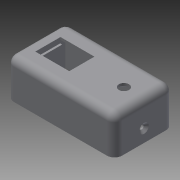
# Autodesk Inventor part: obudowa - timer- front
Saved by Autodesk Inventor 2014 (Build 180170000, 170)
## iProperties
Created: 2018-02-28
Part Number: obudowa - timer- front
Material: Generic
Document SubType Name: Modeling
Designer: HP820
Density: 1 g/cm^3
Appearance: Default
Author: HP820
Autodesk Inventor part; units mm, degrees
ref_plane "YZ Plane" through (0, 0, 0) normal (1, 0, 0) x (0, 1, 0)
ref_plane "XZ Plane" through (0, 0, 0) normal (0, 1, 0) x (-1, 0, 0)
ref_plane "XY Plane" through (0, 0, 0) normal (0, 0, 1) x (1, 0, 0)
sketch "Sketch1" plane through (0, 0, 0) normal (0, 0, 1) x (1, 0, 0)
  line L0 (-40, 20.5) -> (40, 20.5)
  line L1 (40, 20.5) -> (40, -20.5)
  line L2 (40, -20.5) -> (-40, -20.5)
  line L3 (-40, -20.5) -> (-40, 20.5)
  line L4 (-40, 20.5) -> (40, -20.5) construction
  line L5 (40, 20.5) -> (-40, -20.5) construction
  line L6 (-43, 23.5) -> (43, 23.5)
  line L7 (43, 23.5) -> (43, -23.5)
  line L8 (43, -23.5) -> (-43, -23.5)
  line L9 (-43, -23.5) -> (-43, 23.5)
  line L10 (-43, 23.5) -> (43, -23.5) construction
  line L11 (43, 23.5) -> (-43, -23.5) construction
  point P0 (0, 0)
  dimension "d0" = 80
  dimension "d1" = 41
  dimension "d2" = 86
  dimension "d3" = 47
  constraints: 24 end point, 4 midpoint, 4 parallel, 2 horizontal, 2 perpendicular
  measures "d0" distance of L1.end L2.end
  measures "d1" distance of L0.end L1.end
  measures "d2" distance of L7.end L8.end
  measures "d3" distance of L6.end L7.end
extrude "Extrusion1" add sketch "Sketch1" against normal blind 30
sketch "Sketch2" plane through (0, 0, 0) normal (0, 0, 1) x (1, 0, 0)
  line L0 (-40, -20.5) -> (-40, 20.5) projected
  line L1 (-40, 20.5) -> (40, 20.5) projected
  line L2 (40, 20.5) -> (40, -20.5) projected
  line L3 (40, -20.5) -> (-40, -20.5) projected
  point P0 (0, 0)
extrude "Extrusion2" add sketch "Sketch2" against normal blind 3
sketch "Sketch4" plane through (0, 0, 0) normal (0, 0, 1) x (1, 0, 0)
  line L0 (-43, 23.5) -> (43, 23.5) projected
  line L1 (-43, -23.5) -> (-43, 23.5) projected
  line L2 (43, -23.5) -> (-43, -23.5) projected
  line L3 (43, 23.5) -> (43, -23.5) projected
  line L4 (-39.5, 20) -> (39.5, 20)
  line L5 (39.5, 20) -> (39.5, -20)
  line L6 (39.5, -20) -> (-39.5, -20)
  line L7 (-39.5, -20) -> (-39.5, 20)
  line L8 (-39.5, 20) -> (39.5, -20) construction
  line L9 (39.5, 20) -> (-39.5, -20) construction
  point P0 (0, 0)
  dimension "d12" = 79
  dimension "d13" = 40
  constraints: 12 end point, 2 midpoint, 2 parallel, 1 horizontal, 1 perpendicular
  measures "d12" distance of L5.end L6.end
  measures "d13" distance of L4.end L5.end
sketch "Sketch5" plane through (0, 0, 0) normal (0, 0, 1) x (1, 0, 0)
  line L0 (-33.23, 9.75) -> (-6.23, 9.75)
  line L1 (-6.23, 9.75) -> (-6.23, -10.25)
  line L2 (-6.23, -10.25) -> (-33.23, -10.25)
  line L3 (-33.23, -10.25) -> (-33.23, 9.75)
  line L4 (-33.23, 9.75) -> (-6.23, -10.25) construction
  line L5 (-6.23, 9.75) -> (-33.23, -10.25) construction
  line L6 (-39.5, 20) -> (39.5, 20) projected
  line L7 (-39.5, -20) -> (-39.5, 20) projected
  line L8 (39.5, -20) -> (-39.5, -20) projected
  point P0 (0, 0)
  point P1 (-19.73, -0.25)
  dimension "d14" = 27
  dimension "d15" = 20
  dimension "d16" = 10.25
  dimension "d17" = 6.27
  constraints: 12 end point, 2 midpoint, 2 parallel, 1 horizontal, 1 perpendicular
  measures "d14" distance of L1.end L2.end
  measures "d15" distance of L0.end L1.end
  measures "d16" distance between parallel lines of L6 L0
  measures "d17" distance between parallel lines of L7 L3
extrude "Extrusion3" cut sketch "Sketch5" against normal blind 3
sketch "Sketch6" plane through (0, 0, 0) normal (0, 0, 1) x (1, 0, 0)
  circle A0 centre (26.5, 0.5) radius 4
  line L0 (39.5, -20) -> (-39.5, -20) projected
  line L1 (39.5, 20) -> (39.5, -20) projected
  line L2 (-39.5, 20) -> (39.5, 20) projected
  point P0 (0, 0)
  dimension "d20" = 8
  dimension "d21" = 20.5
  dimension "d22" = 13
  constraints: 1 centre point
  measures "d20" diameter of A0
  measures "d21" distance from line of A0.centre L0
  measures "d22" distance from line of A0.centre L1
extrude "Extrusion4" cut sketch "Sketch6" against normal blind 3
chamfer "Chamfer1" distance 1 angle 45 4 edges at (-6.23, -0.25, -3) (-19.73, 9.75, -3) (-19.73, -10.25, -3) (-33.23, -0.25, -3)
chamfer "Chamfer2" distance 1 angle 45 1 edges at (22.5, 0.5, -3)
fillet "Fillet1" radius 6 4 edges at (0, 23.5, 0) (43, 0, 0) (0, -23.5, 0) (-43, 0, 0)
fillet "Fillet2" radius 6 8 edges at (-41.2426, 21.7426, -1.7574) (-43, 23.5, -18) (41.2426, 21.7426, -1.7574) (43, 23.5, -18) (41.2426, -21.7426, -1.7574) (43, -23.5, -18) (-43, -23.5, -18) (-41.2426, -21.7426, -1.7574)
sketch "Sketch7" plane through (-43, -17.5, -6) normal (-1, 0, 0) x (0, 0, 1)
  line L0 (-24, 0) -> (-24, 35) projected
  circle A0 centre (-14, 17.5) radius 1.75
  point P0 (6, 17.5)
  dimension "d33" = 3.5
  dimension "d34" = 10
  constraints: 1 centre point
  measures "d33" diameter of A0
  measures "d34" distance from line of A0.centre L0
extrude "Extrusion5" cut sketch "Sketch7" against normal through all
chamfer "Chamfer3" distance 2 angle 45 2 edges at (-43, 0, -21.75) (43, 0, -21.75)
sketch "Sketch8" plane through (-40, -20.5, -30) normal (1, 0, 0) x (0, 0, -1)
  line L0 (-27, 41) -> (-27, 0) projected
  line L1 (-19, 36.7314) -> (-16, 36.7314)
  line L2 (-16, 36.7314) -> (-16, 4.7314)
  line L3 (-16, 4.7314) -> (-19, 4.7314)
  line L4 (-19, 4.7314) -> (-19, 36.7314)
  point P0 (-30, 20.5)
  dimension "d40" = 3
  dimension "d41" = 32
  dimension "d42" = 8
  constraints: 8 end point, 2 parallel, 1 horizontal, 1 perpendicular
  measures "d40" distance of L2.end L3.end
  measures "d41" distance of L1.end L2.end
  measures "d42" distance between parallel lines of L4 L0
extrude "Extrusion6" add sketch "Sketch8" along normal blind 1.6
sketch "Sketch9" plane through (40, -20.5, -30) normal (-1, 0, 0) x (0, 0, 1)
  line L0 (16, 36.7314) -> (19, 36.7314) projected
  line L1 (19, 36.7314) -> (19, 4.7314) projected
  line L2 (19, 4.7314) -> (16, 4.7314) projected
  line L3 (16, 4.7314) -> (16, 36.7314) projected
  point P0 (30, 20.5)
extrude "Extrusion7" add sketch "Sketch9" along normal blind 1.6
body "Solid1"
